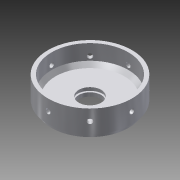
# Autodesk Inventor part: Forward Closure
Saved by Autodesk Inventor 2015 (Build 190159000, 159)
## iProperties
Created: 2015-12-03
Part Number: Forward Closure
Material: Aluminum 6061 T6 0 Cold Formed
Document SubType Name: Modeling
Designer: Jared
Density: 2.7 g/cm^3
Appearance: Aluminum - Flat
Author: Jared
Autodesk Inventor part; units mm, degrees
ref_plane "YZ Plane" through (0, 0, 0) normal (1, 0, 0) x (0, 1, 0)
ref_plane "XZ Plane" through (0, 0, 0) normal (0, 1, 0) x (-1, 0, 0)
ref_plane "XY Plane" through (0, 0, 0) normal (0, 0, 1) x (1, 0, 0)
sketch "Sketch1" plane through (0, 0, 0) normal (0, 0, 1) x (1, 0, 0)
  line L0 (-71.4375, 45.085) -> (-65.0875, 45.085)
  line L1 (-19.05, 0) -> (-19.05, 5.08)
  line L2 (-19.05, 5.08) -> (-22.051, 5.08)
  line L3 (-22.051, 5.08) -> (-22.051, 8.6106)
  line L4 (-22.051, 8.6106) -> (-19.05, 8.6106)
  line L5 (-19.05, 0) -> (-19.05, 5.08)
  line L6 (-19.05, 8.6106) -> (-19.05, 12.7)
  line L7 (0, 0) -> (0, 17.0653)
  line L8 (-71.4375, 6.985) -> (-65.4939, 6.985)
  line L9 (-65.4939, 6.985) -> (-65.4939, 0)
  line L10 (-71.4375, 45.085) -> (-71.4375, 6.985)
  line L11 (-65.4939, 0) -> (-65.4939, -1.27)
  line L12 (-65.4939, -1.27) -> (-19.05, -1.27)
  line L13 (-19.05, -1.27) -> (-19.05, 0)
  line L14 (-65.0875, 19.05) -> (-58.7375, 12.7)
  line L15 (-65.0875, 45.085) -> (-65.0875, 19.05)
  line L16 (-58.7375, 12.7) -> (-19.05, 12.7)
  dimension "d3" = 19.05
  dimension "d8" = 12.7
  dimension "d9" = 5.08
  dimension "d10" = 3.001
  dimension "d11" = 3.5306
  dimension "d12" = 4.0894
  dimension "d26" = 5.9436
  dimension "d28" = 1.27
  dimension "d29" = 6.985
  dimension "d30" = 38.1
  dimension "d31" = 46.4439
  dimension "d32" = 1.27
  dimension "d35" = 39.6875
  dimension "d37" = 135
  dimension "d40" = 71.4375
  dimension "d41" = 20.32
  dimension "d42" = 26.035
  constraints: 34 end point, 10 perpendicular, 3 vertical, 1 horizontal, 1 parallel
  measures "d3" distance of L7.start L1.start
  measures "d8" distance of L1.start L6.end
  measures "d9" distance of L1.start L1.end
  measures "d10" distance of L1.end L2.end
  measures "d11" distance of L2.end L3.end
  measures "d12" distance of L4.end L6.end
  measures "d26" distance of L8.start L8.end
  measures "d28" distance of L9.end L11.end
  measures "d29" distance of L8.end L9.end
  measures "d30" distance of L0.start L8.start
  measures "d31" distance of L11.end L12.end
  measures "d32" distance from line of L7.start L12
  measures "d35" distance of L14.end L6.end
  measures "d37" angle of L16 L14
  measures "d40" distance between parallel lines of L7 L10
  measures "d41" distance from line of L14.start L12
  measures "d42" distance of L0.end L14.start
revolve "Revolution3" add sketch "Sketch1" angle 360 about axis through (0, 0, 0) along (0, 1, 0)
sketch "Sketch2" plane through (0, 0, 0) normal (1, 0, 0) x (0, 1, 0)
  line L0 (45.085, -65.0875) -> (45.085, 65.0875) projected
  circle A0 centre (26.035, 0) radius 3.9688
  point P0 (0, 0)
  dimension "d45" = 7.9375
  constraints: 1 centre point
  measures "d45" diameter of A0
extrude "Extrusion1" cut sketch "Sketch2" along normal blind 207.9625
pattern_circular "Circular Pattern1" count 8 over 360 about axis through (0, 32.0675, 0) along (0, 1, 0) of "Extrusion1"
body "Solid3"
